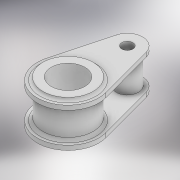
# Autodesk Inventor part: 零件1
Saved by Autodesk Inventor 2020 (Build 240168000, 168)
## iProperties
Created: 2021-03-24
Part Number: 零件1
Material: 常规
Document SubType Name: Modeling
Designer: Luorily
Density: 1 g/cm^3
Appearance: 默认
Author: Luorily
Autodesk Inventor part; units mm, degrees
ref_plane "YZ Plane" through (0, 0, 0) normal (1, 0, 0) x (0, 1, 0)
ref_plane "XZ Plane" through (0, 0, 0) normal (0, 1, 0) x (-1, 0, 0)
ref_plane "XY Plane" through (0, 0, 0) normal (0, 0, 1) x (1, 0, 0)
sketch "草图1" plane through (0, 0, 0) normal (0, 1, 0) x (-1, 0, 0)
  circle A0 centre (0, 0) radius 30
  circle A1 centre (0, 0) radius 45
  circle A2 centre (0, -106) radius 10
  circle A3 centre (0, 0) radius 55
  arc A4 (-26.5584, -113.1344) -> (26.5584, -113.1344) centre (0, -106) ccw
  line L0 (53.1168, -14.2689) -> (26.5584, -113.1344)
  line L1 (-53.1168, -14.2689) -> (-26.5584, -113.1344)
  circle A5 centre (0, -106) radius 20
  dimension "d0" = 60
  dimension "d1" = 90
  dimension "d3" = 20
  dimension "d4" = 110
  dimension "d5" = 55
  dimension "d8" = 40
  constraints: 6 centre point, 5 coincident, 4 end point, 4 point on circle, 4 tangent
  measures "d0" diameter of A0
  measures "d1" diameter of A1
  measures "d3" diameter of A2
  measures "d4" diameter of A3
  measures "d5" diameter of A4
  measures "d8" diameter of A5
extrude "拉伸2" add sketch "草图1" along normal blind 70 contours A5
extrude "拉伸3" add sketch "草图1" along normal blind 75 and the other way blind 5 contours A1
extrude "拉伸4" add sketch "草图1" along normal blind 8 contours A3 | A3 L0 A4 L1
sketch "草图2" plane through (0, 70, -106) normal (0, 1, 0) x (1, 0, 0)
  circle A0 centre (0, 0) radius 20 projected
  circle A1 centre (0, 0) radius 10 projected
  arc A2 (26.5584, 7.1344) -> (-26.5584, 7.1344) centre (0, 0) ccw
  arc A3 (-53.1168, -91.7311) -> (53.1168, -91.7311) centre (0, -106) ccw
  line L0 (53.1168, -91.7311) -> (26.5584, 7.1344) projected
  line L1 (26.5584, 7.1344) -> (53.1168, -91.7311)
  line L2 (-26.5584, 7.1344) -> (-53.1168, -91.7311) projected
  line L3 (-26.5584, 7.1344) -> (-53.1168, -91.7311)
  circle A4 centre (0, -106) radius 30
  circle A5 centre (0, 0) radius 10
  dimension "d19" = 60
  constraints: 5 point on circle, 4 centre point, 4 coincident, 4 end point, 2 tangent
  measures "d19" diameter of A4
extrude "拉伸5" add sketch "草图2" against normal blind 8 contours L0 A3 L2 A2
fillet "圆角1" radius 5 4 edges at (45, 70, 0) (45, 0, 0) (45, 62, 0) (45, 8, 0)
